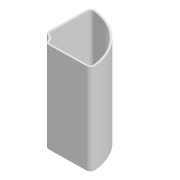
# Autodesk Inventor part: 桶
Saved by Autodesk Inventor 2021 (Build 250183000, 183)
## iProperties
Created: 2024-06-10
Part Number: 桶
Material: 常规
Document SubType Name: Modeling
Designer: 86155
Density: 1 g/cm^3
Appearance: 默认
Author: 86155
Autodesk Inventor part; units mm, degrees
ref_plane "YZ Plane" through (0, 0, 0) normal (1, 0, 0) x (0, 1, 0)
ref_plane "XZ Plane" through (0, 0, 0) normal (0, 1, 0) x (-1, 0, 0)
ref_plane "XY Plane" through (0, 0, 0) normal (0, 0, 1) x (1, 0, 0)
sketch "草图1" plane through (0, 0, 0) normal (0, 1, 0) x (-1, 0, 0)
  circle A0 centre (0, 0) radius 650
  arc A1 (-64.9652, -596.4726) -> (-9.5591, -547.6391) centre (-59.5515, -546.7665) ccw projected
  line L0 (-2.4681, -141.3998) -> (-9.5591, -547.6391) projected
  arc A2 (-2.4681, -141.3998) -> (-34.9737, -93.6848) centre (-52.4605, -140.5272) ccw projected
  arc A3 (-93.6848, -34.9737) -> (-34.9737, -93.6848) centre (0, 0) ccw projected
  arc A4 (-93.6848, -34.9737) -> (-141.3998, -2.4681) centre (-140.5272, -52.4605) ccw projected
  line L1 (-547.6391, -9.5591) -> (-141.3998, -2.4681) projected
  arc A5 (-547.6391, -9.5591) -> (-596.4726, -64.9652) centre (-546.7665, -59.5515) ccw projected
  arc A6 (-596.4726, -64.9652) -> (-64.9652, -596.4726) centre (0, 0) ccw projected
  arc A7 (-64.9652, -596.4726) -> (-9.5591, -547.6391) centre (-59.5515, -546.7665) ccw
  line L2 (-9.5591, -547.6391) -> (-2.4681, -141.3998)
  arc A8 (-2.4681, -141.3998) -> (-34.9737, -93.6848) centre (-52.4605, -140.5272) ccw
  arc A9 (-93.6848, -34.9737) -> (-34.9737, -93.6848) centre (0, 0) ccw
  arc A10 (-93.6848, -34.9737) -> (-141.3998, -2.4681) centre (-140.5272, -52.4605) ccw
  line L3 (-141.3998, -2.4681) -> (-547.6391, -9.5591)
  arc A11 (-547.6391, -9.5591) -> (-596.4726, -64.9652) centre (-546.7665, -59.5515) ccw
  arc A12 (-596.4726, -64.9652) -> (-64.9652, -596.4726) centre (0, 0) ccw
  line L4 (-22.4651, -141.0508) -> (-29.556, -547.2901)
  arc A13 (-62.7997, -576.5901) -> (-29.556, -547.2901) centre (-59.5515, -546.7665) ccw
  arc A14 (-576.5901, -62.7997) -> (-62.7997, -576.5901) centre (0, 0) ccw
  arc A15 (-547.2901, -29.556) -> (-576.5901, -62.7997) centre (-546.7665, -59.5515) ccw
  line L5 (-547.2901, -29.556) -> (-141.0508, -22.4651)
  arc A16 (-112.4218, -41.9684) -> (-141.0508, -22.4651) centre (-140.5272, -52.4605) ccw
  arc A17 (-112.4218, -41.9684) -> (-41.9684, -112.4218) centre (0, 0) ccw
  arc A18 (-22.4651, -141.0508) -> (-41.9684, -112.4218) centre (-52.4605, -140.5272) ccw
  dimension "d0" = 1300
  dimension "d3" = 0
  dimension "d4" = 20
  constraints: 24 point on circle, 13 centre point, 8 end point, 1 coincident, 14 other
  measures "d0" diameter of A0
  measures "d3" radial gap between concentric circles of A6 A12
  measures "d4" distance between parallel lines of L2 L4
extrude "拉伸2" add sketch "草图1" along normal blind 1000 contours A6 A5 L1 A4 A3 A2 L0 A1
extrude "拉伸3" add sketch "草图1" along normal blind 30 contours L4 A13 A14 A15 L5 A16 A17 A18
fillet "圆角1" radius 10 8 edges at (569.2726, 30, -39.7152) (344.1704, 30, -26.0106) (123.6368, 30, -27.6671) (84.8528, 30, -84.8528) (27.6671, 30, -123.6368) (26.0106, 30, -344.1704) (39.7152, 30, -569.2726) (410.1219, 30, -410.1219)
